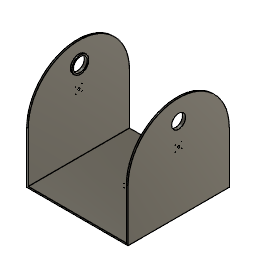
Altitude Baseplate (Autodesk Fusion 360 design; units mm, degrees)
part number: 2026-04-09-23-56-47-011
Autodesk Fusion 360 part; units mm, degrees
sketch "Sketch1" plane through (0, 0, 0) normal (0, 0, 1) x (1, 0, 0)
  line L0 (0, 0) -> (500, 0)
  line L1 (500, 0) -> (500, 500)
  line L2 (500, 500) -> (0, 500)
  line L3 (0, 500) -> (0, 0)
  circle A0 centre (250, 250) radius 1.5
  circle A1 centre (230, 249.99) radius 1.5
  circle A2 centre (270, 250.01) radius 1.5
  circle A3 centre (249.99, 270) radius 1.5
  circle A4 centre (250.01, 230) radius 1.5
  point P0 (250.01, 230)
  point P1 (270, 250.01)
  point P2 (249.99, 270)
  dimension "d1" = 500
  dimension "d2" = 500
  dimension "d3" = 3
  dimension "d4" = 250
  dimension "d5" = 250
  dimension "d50" = 3
  dimension "d52" = 360
  dimension "d53" = 20
  dimension "d54" = 0.01
  dimension "d55" = 3
  dimension "d56" = 3
  dimension "d57" = 3
  constraint horizontal L0
  constraint vertical L1
  constraint horizontal L2
  constraint vertical L3
  constraint coincident L0.start L3.end
  constraint coincident P1 A2.centre
  constraint coincident P2 A3.centre
  constraint coincident P0 A4.centre
  measures "d1" distance of L1.end L2.end
  measures "d2" distance of L0.start L2.end
  measures "d3" diameter of A0
  measures "d4" distance of L3 A0.centre
  measures "d5" distance of L2 A0.centre
  measures "d50" diameter of A1
  measures "d53" horizontal distance of A0.centre A1.centre
  measures "d54" vertical distance of A0.centre A1.centre
  measures "d55" diameter of A2
  measures "d56" diameter of A3
  measures "d57" diameter of A4
extrude "Extrude1" add sketch "Sketch1" along normal blind 7.5
sketch "Sketch2" plane through (0, 0, 7.5) normal (0, 0, 1) x (-1, 0, 0)
  circle A0 centre (-250, -250) radius 1.5
  line L0 (0, -500) -> (0, 0)
  line L1 (0, 0) -> (-500, 0)
  line L2 (-500, 0) -> (-500, -500)
  line L3 (-500, -500) -> (0, -500)
  line L4 (0, -500) -> (-7.5, -500)
  line L5 (-7.5, -500) -> (-7.5, 0)
  line L6 (-7.5, 0) -> (0, 0)
  line L7 (0, 0) -> (0, -500)
  line L8 (-500, -500) -> (-492.5, -500)
  line L9 (-492.5, -500) -> (-492.5, 0)
  line L10 (-492.5, 0) -> (-500, 0)
  line L11 (-500, 0) -> (-500, -500)
  circle A1 centre (-270, -250.01) radius 1.5
  circle A2 centre (-249.99, -270) radius 1.5
  circle A3 centre (-230, -249.99) radius 1.5
  circle A4 centre (-250.01, -230) radius 1.5
  dimension "d8" = 7.5
  dimension "d9" = 7.5
  constraint horizontal L4
  constraint vertical L5
  constraint horizontal L6
  constraint vertical L7
  constraint coincident L1 L5.end
  constraint coincident L0.start L3.end
  constraint horizontal L8
  constraint vertical L9
  constraint horizontal L10
  constraint vertical L11
  constraint coincident L1 L9.end
  constraint coincident L2.end L3.start
  measures "d8" distance of L5 L7
  measures "d9" distance of L9 L11
extrude "Extrude2" add sketch "Sketch2" along normal blind 500 contours L0 L1 L3 L4 L5 L6 L7 | L1 L2 L3 L8 L9 L10 L11
fillet "Fillet1" radius 250 1 edges at (3.75, 500, 507.5)
fillet "Fillet2" radius 250 1 edges at (3.75, 0, 507.5)
fillet "Fillet3" radius 250 1 edges at (496.25, 500, 507.5)
fillet "Fillet4" radius 250 1 edges at (496.25, 0, 507.5)
sketch "Sketch3" plane through (0, 0, 0) normal (-1, 0, 0) x (0, -1, 0)
  arc A0 (0, 257.5) -> (-500, 257.5) centre (-250, 257.5) ccw
  line L0 (-500, 257.5) -> (-500, 0)
  line L1 (-500, 0) -> (0, 0)
  line L2 (0, 0) -> (0, 257.5)
  circle A1 centre (-250, 407.5) radius 34
  dimension "d20" = 68
  dimension "d22" = 250
  measures "d20" diameter of A1
  measures "d22" distance of L0 A1.centre
hole "Hole1" at (0, 250, 407.5) direction (1, 0, 0) diameter 68 depth 6000 tip angle 118
sketch "Sketch4" plane through (7.5, 0, 0) normal (1, 0, 0) x (0, 1, 0)
  circle A0 centre (250, 407.5) radius 34
  arc A1 (500, 257.5) -> (0, 257.5) centre (250, 257.5) ccw
  line L0 (0, 257.5) -> (0, 7.5)
  line L1 (0, 7.5) -> (500, 7.5)
  line L2 (500, 7.5) -> (500, 257.5)
  circle A2 centre (250, 407.5) radius 41.5
  dimension "d26" = 7.5
extrude "Extrude3" add sketch "Sketch4" along normal blind 7.5 contours A2
sketch "Sketch5" plane through (492.5, 0, 0) normal (-1, 0, 0) x (0, -1, 0)
  circle A0 centre (-250, 407.5) radius 34
  arc A1 (0, 257.5) -> (-500, 257.5) centre (-250, 257.5) ccw
  line L0 (-500, 257.5) -> (-500, 7.5)
  line L1 (-500, 7.5) -> (0, 7.5)
  line L2 (0, 7.5) -> (0, 257.5)
  circle A2 centre (-250, 407.5) radius 41.5
  dimension "d29" = 7.5
extrude "Extrude4" add sketch "Sketch5" along normal blind 7.5 contours A2
sketch "Sketch6" plane through (500, 0, 0) normal (1, 0, 0) x (0, 1, 0)
  circle A0 centre (250, 407.5) radius 34
  arc A1 (500, 257.5) -> (0, 257.5) centre (250, 257.5) ccw
  line L0 (0, 257.5) -> (0, 0)
  line L1 (0, 0) -> (500, 0)
  line L2 (500, 0) -> (500, 257.5)
  circle A2 centre (250, 298.7) radius 5.625
  circle A3 centre (234.5, 314.2) radius 1.55
  circle A4 centre (265.5, 314.2) radius 1.55
  circle A5 centre (265.5, 283.2) radius 1.55
  circle A6 centre (234.5, 283.2) radius 1.55
  dimension "d32" = 11.25
  dimension "d33" = 108.8
  dimension "d37" = 298.7
  dimension "d38" = 15.5
  dimension "d39" = 15.5
  dimension "d40" = 15.5
  dimension "d41" = 15.5
  dimension "d42" = 15.5
  dimension "d43" = 15.5
  dimension "d44" = 15.5
  dimension "d45" = 15.5
  dimension "d46" = 3.1
  dimension "d47" = 3.1
  dimension "d48" = 3.1
  dimension "d49" = 3.1
  measures "d32" diameter of A2
  measures "d33" distance of A0.centre A2.centre
  measures "d37" distance of L1 A2.centre
  measures "d38" vertical distance of A2.centre A6.centre
  measures "d39" horizontal distance of A2.centre A6.centre
  measures "d40" vertical distance of A2.centre A3.centre
  measures "d41" horizontal distance of A2.centre A3.centre
  measures "d42" horizontal distance of A2.centre A4.centre
  measures "d43" vertical distance of A2.centre A4.centre
  measures "d44" vertical distance of A2.centre A5.centre
  measures "d45" horizontal distance of A2.centre A5.centre
  measures "d46" diameter of A3
  measures "d47" diameter of A4
  measures "d48" diameter of A5
  measures "d49" diameter of A6
extrude "Extrude5" cut sketch "Sketch6" against normal blind 700 contours A2 | A3 | A4 | A5 | A6
equation "d37 = 407.5 mm - 108.8 mm"
equation "d38 = ( 31 / 2 ) * 1 mm"
equation "d39 = ( 31 / 2 ) * 1 mm"
equation "d40 = ( 31 / 2 ) * 1 mm"
equation "d41 = ( 31 / 2 ) * 1 mm"
equation "d42 = ( 31 / 2 ) * 1 mm"
equation "d43 = ( 31 / 2 ) * 1 mm"
equation "d44 = ( 31 / 2 ) * 1 mm"
equation "d45 = ( 31 / 2 ) * 1 mm"
